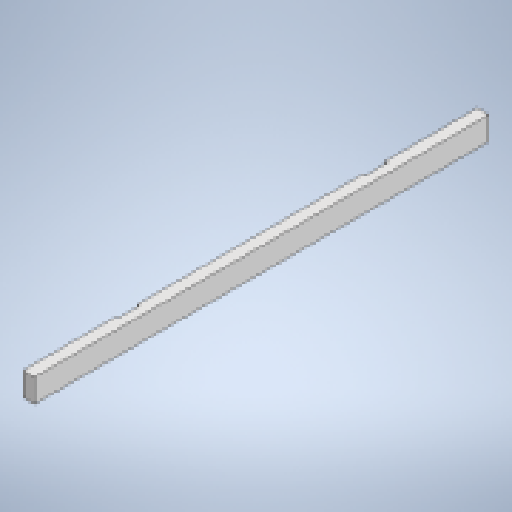
# Autodesk Inventor part: side_panel
Saved by Autodesk Inventor 2025.2 (Build 292293000, 293)
## iProperties
Created: 2025-01-19
Part Number: side_panel
Material: Типовые
Document SubType Name: Modeling
Designer: Admin
Density: 1 g/cm^3
Appearance: По умолчанию
Author: Admin
Autodesk Inventor part; units mm, degrees
ref_plane "YZ Plane" through (0, 0, 0) normal (1, 0, 0) x (0, 1, 0)
ref_plane "XZ Plane" through (0, 0, 0) normal (0, 1, 0) x (-1, 0, 0)
ref_plane "XY Plane" through (0, 0, 0) normal (0, 0, 1) x (1, 0, 0)
sketch "Эскиз1" plane through (0, 0, 0) normal (1, 0, 0) x (0, 1, 0)
  line L0 (-50, -978) -> (50, -978)
  line L1 (50, -978) -> (50, 978)
  line L2 (50, 978) -> (-50, 978)
  line L3 (-50, 978) -> (-50, -978)
  line L4 (-50, -978) -> (50, 978) construction
  line L5 (50, -978) -> (-50, 978) construction
  point P0 (0, 0)
  dimension "d0" = 100
  dimension "d1" = 1956
  constraints: 12 end point, 2 midpoint, 2 parallel, 1 horizontal, 1 perpendicular
  measures "d0" distance of L2.end L1.end
  measures "d1" distance of L1.end L0.end
extrude "Выдавливание1" add sketch "Эскиз1" along normal blind 50
sketch "Эскиз2" plane through (0, 50, 978) normal (0, 1, 0) x (1, 0, 0)
  line L0 (0, 1556) -> (10, 1556)
  line L1 (10, 1463) -> (0, 1463)
  line L2 (10, 1463) -> (10, 1556)
  line L3 (0, 1556) -> (0, 1463)
  point P0 (0, 978)
  constraints: 8 end point
extrude "Выдавливание2" cut sketch "Эскиз2" against normal blind 55
sketch "Эскиз3" plane through (0, 50, 978) normal (0, 1, 0) x (1, 0, 0)
  line L0 (10, 493) -> (-0.0484, 493)
  line L1 (0, 400) -> (10, 400)
  line L2 (10, 400) -> (10, 493)
  line L3 (-0.0484, 493) -> (0, 400)
  point P0 (0, 978)
  constraints: 8 end point
extrude "Выдавливание3" cut sketch "Эскиз3" against normal blind 29
